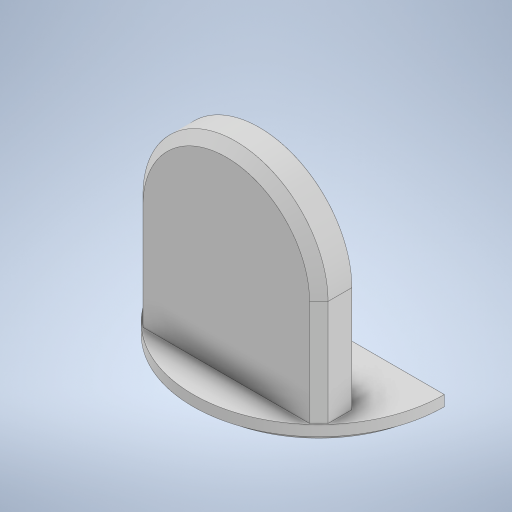
# Autodesk Inventor part: Base 1 right
Saved by Autodesk Inventor 2023 (Build 270158000, 158)
## iProperties
Created: 2024-06-28
Part Number: Base 1 right
Material: Generic
Document SubType Name: Modeling
Designer: Swoby
Density: 1 g/cm^3
Appearance: Default
Author: Swoby
Autodesk Inventor part; units mm, degrees
ref_plane "YZ Plane" through (0, 0, 0) normal (1, 0, 0) x (0, 1, 0)
ref_plane "XZ Plane" through (0, 0, 0) normal (0, 1, 0) x (-1, 0, 0)
ref_plane "XY Plane" through (0, 0, 0) normal (0, 0, 1) x (1, 0, 0)
sketch "Sketch1" plane through (0, 0, 0) normal (0, 0, 1) x (1, 0, 0)
  circle A0 centre (0, 0) radius 35
  line L0 (-35, 0) -> (-35, -40)
  line L1 (-35, -40) -> (35, -40)
  line L2 (35, -40) -> (35, 0)
  dimension "d0" = 70
  dimension "d1" = 40
  constraints: 6 end point, 2 point on circle, 2 tangent, 1 centre point, 1 coincident, 1 parallel, 1 perpendicular, 1 vertical
  measures "d0" diameter of A0
  measures "d1" distance of L1.end L2.end
extrude "Extrusion1" add sketch "Sketch1" along normal blind 12.5
sketch "Sketch2" plane through (-35, -40, 0) normal (0, -1, 0) x (1, 0, 0)
  arc A0 (82.5, -22.5) -> (-12.5, -22.5) centre (35, -22.5) ccw
  line L0 (0, 12.5) -> (70, 12.5) construction
  line L1 (35, 12.5) -> (35, 0)
  line L2 (82.5, -22.5) -> (-12.5, -22.5)
  arc A1 (-12.5, -22.5) -> (82.5, -22.5) centre (35, -22.5) ccw construction
  dimension "d4" = 95
  dimension "d6" = 35
  constraints: 4 end point, 4 point on circle, 2 centre point, 2 midpoint, 1 parallel, 1 point on line, 1 vertical
  measures "d4" diameter of A0
  measures "d6" distance from line of L0 A0.centre
extrude "Extrusion2" add sketch "Sketch2" along normal blind 8
chamfer "Chamfer1" distance 3.5 angle 45 3 edges at (0, 35, 12.5) (-35, -20, 12.5) (35, -20, 12.5)
sketch "Sketch3" plane through (0, 0, 0) normal (0, 0, -1) x (-1, 0, 0)
  circle A0 centre (0, 0) radius 12.5
  dimension "d12" = 25
  constraints: 1 centre point, 1 coincident
  measures "d12" diameter of A0
extrude "Extrusion3" cut sketch "Sketch3" against normal blind 7
sketch "Sketch4" plane through (-35, -48, 0) normal (0, -1, 0) x (1, 0, 0)
  arc A0 (82.5, -22.5) -> (-12.5, -22.5) centre (35, -22.5) ccw projected
  arc A1 (77.5, -22.5) -> (-7.5, -22.5) centre (35, -22.5) ccw
  arc A2 (82.5, -22.5) -> (-12.5, -22.5) centre (35, -22.5) ccw projected
  line L0 (-7.5, -22.5) -> (-12.5, -22.5)
  line L1 (82.5, -22.5) -> (77.5, -22.5)
  line L2 (-12.5, -22.5) -> (82.5, -22.5) projected
  circle A3 centre (35, -22.5) radius 32.5
  circle A4 centre (35, -22.5) radius 30
  point P0 (35, 0)
  point P1 (5, -22.5)
  point P2 (65, -22.5)
  point P3 (67.5, -22.5)
  point P4 (2.5, -22.5)
  dimension "d16" = 5
  dimension "d20" = 65
  dimension "d21" = 60
  constraints: 4 coincident, 4 end point, 3 centre point, 2 point on circle, 1 collinear
  measures "d16" radial gap between concentric circles of A0 A1
  measures "d20" diameter of A3
  measures "d21" diameter of A4
extrude "Extrusion4" cut sketch "Sketch4" against normal blind 4 contours L1 A1 L0 A0 | L2 A4 A3 picked at (43.6934, 7.7339)
body "Solid1"
